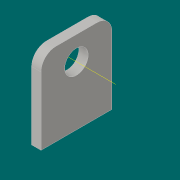
# Autodesk Inventor part: Ell-Tab_small
Saved by Autodesk Inventor 2016 (Build 200138000, 138)
## iProperties
Created: 2017-02-21
Part Number: Ell-Tab_small
Material: Generic
Document SubType Name: Modeling
Designer: katzchristy
Density: 1 g/cm^3
Appearance: Default
Author: katzchristy
Autodesk Inventor part; units mm, degrees
ref_plane "YZ Plane" through (0, 0, 0) normal (1, 0, 0) x (0, 1, 0)
ref_plane "XZ Plane" through (0, 0, 0) normal (0, 1, 0) x (-1, 0, 0)
ref_plane "XY Plane" through (0, 0, 0) normal (0, 0, 1) x (1, 0, 0)
sketch "Sketch1" plane through (0, 0, 0) normal (1, 0, 0) x (0, 1, 0)
  circle A0 centre (0, 0) radius 2.54
  line L0 (5.08, 7.62) -> (-12.7, 7.62)
  line L1 (-12.7, 7.62) -> (-12.7, -7.62)
  line L2 (-12.7, -7.62) -> (5.08, -7.62)
  line L3 (5.08, -7.62) -> (5.08, 7.62)
  point P0 (5.08, 0)
  dimension "d0" = 5.08
  dimension "d1" = 15.24
  dimension "d2" = 17.78
  dimension "d5" = 5.08
  constraints: 8 end point, 2 parallel, 1 centre point, 1 coincident, 1 horizontal, 1 horizontal alignment, 1 midpoint, 1 perpendicular
  measures "d0" diameter of A0
  measures "d1" distance of L2.end L0.start
  measures "d2" distance of L1.end L2.end
  measures "d5" distance from line of L3 point (0, 0)
extrude "Extrusion1" add sketch "Sketch1" along normal blind 2.032
fillet "Fillet1" radius 3.175 2 edges at (1.016, 5.08, 7.62) (1.016, 5.08, -7.62)
body "Solid1"
